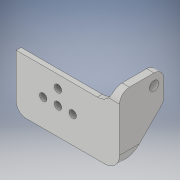
# Autodesk Inventor part: tibia_vFINAL
Saved by Autodesk Inventor 2019 (Build 230136000, 136)
## iProperties
Created: 2019-01-20
Part Number: tibia_vFINAL
Material: Generic
Document SubType Name: Modeling
Designer: Daniel
Density: 1 g/cm^3
Appearance: Default
Author: Daniel
Autodesk Inventor part; units mm, degrees
ref_plane "YZ Plane" through (0, 0, 0) normal (1, 0, 0) x (0, 1, 0)
ref_plane "XZ Plane" through (0, 0, 0) normal (0, 1, 0) x (-1, 0, 0)
ref_plane "XY Plane" through (0, 0, 0) normal (0, 0, 1) x (1, 0, 0)
sketch "Sketch1" plane through (0, 0, 0) normal (0, 1, 0) x (-1, 0, 0)
  line L0 (39, 2) -> (-3, 2)
  line L1 (-3, 2) -> (-3, 0)
  line L2 (-3, 0) -> (39, 0)
  line L3 (39, 0) -> (39, 2)
  line L4 (47.4, 0) -> (-11.4, 0) projected
  line L5 (0, -19.6) -> (0, 5.6) projected
  line L6 (0, -16) -> (-3, -16)
  line L7 (-3, -16) -> (-3, 0)
  line L8 (-3, 0) -> (0, 0)
  line L9 (0, 0) -> (0, -16)
  point P0 (0, 0)
  dimension "d0" = 2
  dimension "d1" = 3
  dimension "d2" = 42
  dimension "d3" = 18
  constraints: 16 end point, 4 collinear, 4 parallel, 2 horizontal, 2 perpendicular
  measures "d0" distance between parallel lines of L0 L2
  measures "d1" distance between parallel lines of L7 L9
  measures "d2" distance between parallel lines of L1 L3
  measures "d3" distance between parallel lines of L0 L6
extrude "Extrusion1" add sketch "Sketch1" along normal blind 22
sketch "Sketch2" plane through (-39, 0, 2) normal (0, 0, 1) x (1, 0, 0)
  line L0 (0, 0) -> (42, 0) projected
  line L1 (42, 0) -> (42, 22) projected
  line L2 (0, 22) -> (42, 22) projected
  line L3 (0, 0) -> (0, 22) projected
  point P0 (39, 0)
  point P1 (17, 11)
  point P2 (17, 17)
  point P3 (11, 11)
  point P4 (23, 11)
  dimension "d6" = 5
  dimension "d7" = 6
  dimension "d8" = 6
  dimension "d9" = 6
  dimension "d11" = 11
  dimension "d12" = 6
  dimension "d14" = 6
  dimension "d15" = 6
  measures "d6" distance from line of L2 point (17, 17)
  measures "d7" distance of point (17, 11) point (17, 17)
  measures "d8" distance of point (17, 11) point (11, 11)
  measures "d9" distance of point (17, 11) point (23, 11)
  measures "d11" distance from line of L3 point (11, 11)
  measures "d12" horizontal distance of point (17, 17) point (11, 11)
  measures "d14" horizontal distance of point (17, 17) point (23, 11)
  measures "d15" horizontal distance of point (11, 11) point (17, 17)
hole "Hole1" at (-22, 11, 2) at (-22, 17, 2) at (-28, 11, 2) at (-16, 11, 2) direction (0, 0, -1) diameter 3 end through all
sketch "Sketch3" plane through (0, 22, 0) normal (0, 1, 0) x (1, 0, 0)
  line L0 (3, 16) -> (0, 16) projected
  line L1 (0, 16) -> (0, 0) projected
  line L2 (0, 0) -> (-39, 0) projected
  line L3 (-39, 0) -> (-39, -2) projected
  line L4 (-39, -2) -> (3, -2) projected
  line L5 (3, -2) -> (3, 16) projected
  line L6 (0, -2) -> (3, -2)
  line L7 (3, -2) -> (3, 16)
  line L8 (3, 16) -> (0, 16)
  line L9 (0, 16) -> (0, -2)
  line L10 (0, 16) -> (0, 0) projected
  line L11 (3, 16) -> (0, 16) projected
  line L12 (-39, -2) -> (3, -2) projected
  line L13 (3, -2) -> (3, 16) projected
  constraints: 8 end point, 4 collinear, 2 parallel, 1 horizontal, 1 perpendicular
extrude "Extrusion2" add sketch "Sketch3" along normal blind 6 contours L5 L4 L9 L1 L0
sketch "Sketch5" plane through (0, 22, 2) normal (-1, 0, 0) x (0, 0, 1)
  line L0 (0, -22) -> (0, 0) projected
  line L1 (-2, 0) -> (0, 0) projected
  point P0 (-2, -22)
  point P1 (-14, 1.5)
  dimension "d52" = 14
  dimension "d53" = 1.5
  measures "d52" distance from line of L0 point (-14, 1.5)
  measures "d53" distance from line of L1 point (-14, 1.5)
hole "Hole3" at (0, 23.5, -12) direction (1, 0, 0) diameter 3.75 end through all
chamfer "Chamfer3" distance 16 angle 45 1 edges at (1.5, 0, -16)
fillet "Fillet11" radius 4 4 edges at (0, 11, 0) (1.5, 16, -16) (1.5, 28, -16) (1.5, 28, 2)
fillet "Fillet12" radius 6 2 edges at (0, 22, -2) (0, 22, 1)
fillet "Fillet13" radius 6 1 edges at (3, 0, 1)
fillet "Fillet14" radius 4 1 edges at (-39, 0, 1)
body "Solid1"
